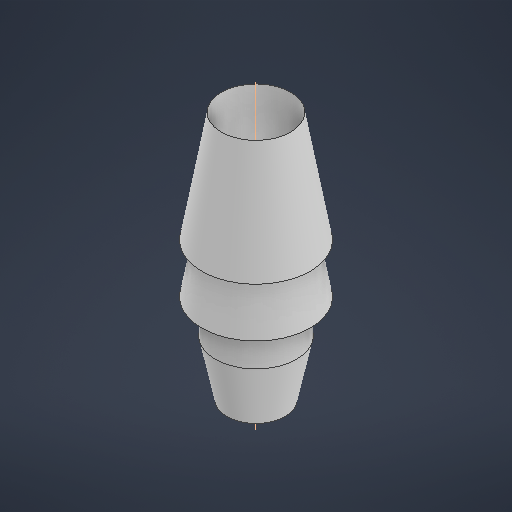
# Autodesk Inventor part: eigthinch
Saved by Autodesk Inventor 2026.2 (Build 302298010, 298A)
## iProperties
Created: 2026-03-08
Part Number: eigthinch
Material: Generic
Document SubType Name: Modeling
Designer: david
Density: 1 g/cm^3
Appearance: Default
Author: david
Autodesk Inventor part; units mm, degrees
ref_plane "YZ Plane" through (0, 0, 0) normal (1, 0, 0) x (0, 1, 0)
ref_plane "XZ Plane" through (0, 0, 0) normal (0, 1, 0) x (-1, 0, 0)
ref_plane "XY Plane" through (0, 0, 0) normal (0, 0, 1) x (1, 0, 0)
sketch "Sketch1" plane through (0, 0, 0) normal (0, 0, 1) x (1, 0, 0)
  line L0 (1.5875, 0) -> (1.5875, 8.89)
  line L1 (1.5875, 8.89) -> (2.4832, 3.81)
  line L2 (1.5875, 8.89) -> (6.7459, 8.89) construction
  line L3 (2.4832, 3.81) -> (2.085, 3.81)
  line L4 (2.085, 3.81) -> (2.4832, 1.5517)
  line L5 (2.4832, 1.5517) -> (1.8611, 1.5517)
  line L6 (1.8611, 1.5517) -> (1.8611, 0)
  line L7 (1.8611, 0) -> (1.5875, 0)
  line L8 (0, -4.826) -> (0, 11.176) projected
  line L9 (1.5875, 0) -> (1.8611, 0)
  line L10 (1.8611, 0) -> (1.8611, -2.54) construction
  line L11 (1.8611, -2.54) -> (1.5875, -2.54) construction
  line L12 (1.5875, -2.54) -> (1.5875, 0) construction
  line L13 (1.5875, 0) -> (1.0583, -2.54)
  line L14 (1.0583, -2.54) -> (1.5875, -2.54) construction
  line L15 (1.8611, 0) -> (1.3319, -2.54)
  line L16 (1.0583, -2.54) -> (1.3319, -2.54)
  point P0 (0, 0)
  point P1 (2.1722, 1.5517)
  dimension "d1" = 1.5875
  dimension "d3" = 0
  dimension "d4" = 80
  dimension "d5" = 0.3982
  dimension "d6" = 2.2583
  dimension "d7" = 1.5517
  dimension "d8" = 1.8611
  dimension "d10" = 8.89
  dimension "d11" = 2.54
  dimension "d12" = 0.2736
  dimension "d17" = 0.2736
  dimension "d18" = 1.0583
  constraints: 32 end point, 5 horizontal, 4 parallel, 3 perpendicular, 1 equal length, 1 midpoint, 1 point on line, 1 vertical
  measures "d1" distance from line of point (0, 0) L0
  measures "d3" vertical distance of point (0, 0) L0.start
  measures "d4" angle of L1 L2
  measures "d5" distance of L1.end L3.end
  measures "d6" distance between parallel lines of L5 L3
  measures "d7" vertical distance of point (0, 0) point (2.172, 1.552)
  measures "d8" distance from line of point (0, 0) L6
  measures "d10" distance of L0.start L0.end
  measures "d11" distance of L9.end L10.end
  measures "d12" distance between parallel lines of L12 L10
  measures "d17" distance of L13.end L15.end
  measures "d18" horizontal distance of point (0, 0) L13.end
revolve "Revolution2" add sketch "Sketch1" angle 360 about axis through (0, -10, 0) along (0, 1, 0)
body "Solid2"
